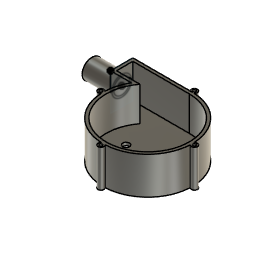
Bottom v3 (Autodesk Fusion 360 design; units mm, degrees)
Autodesk Fusion 360 part; units mm, degrees
sketch "Skizze1" plane through (0, 0, 0) normal (0, 0, 1) x (1, 0, 0)
  circle A0 centre (0, 0) radius 30
  circle A1 centre (0, 0) radius 3
  line L0 (0, 0) -> (14.5, 0)
  circle A2 centre (14.5, 0) radius 2.25
  line L1 (0, 0) -> (-14.5, 0)
  circle A3 centre (-14.5, 0) radius 2.25
  circle A4 centre (-31.5, 0) radius 1
  circle A5 centre (-31.5, 0) radius 2
  circle A6 centre (31.5, 0) radius 1
  circle A7 centre (31.5, 0) radius 2
  circle A8 centre (0, -31.5) radius 1
  circle A9 centre (0, -31.5) radius 2
  circle A10 centre (0, 31.5) radius 1
  circle A11 centre (0, 31.5) radius 2
  line L2 (0, 30) -> (-40, 30)
  line L3 (-40, 30) -> (-40, 15)
  line L4 (-40, 15) -> (0, 15)
  line L5 (0, 15) -> (0, 30)
  line L6 (-40, 30) -> (-40, 28)
  line L7 (-40, 28) -> (0, 28)
  circle A12 centre (0, 0) radius 28
  line L8 (-40, 15) -> (-40, 17)
  line L9 (-40, 17) -> (0, 17)
  line L10 (-38, 28) -> (-38, 17)
  dimension "d1" = 60
  dimension "d2" = 6
  dimension "d3" = 14.5
  dimension "d4" = 4.5
  dimension "d5" = 14.5
  dimension "d6" = 4.5
  dimension "d7" = 2
  dimension "d8" = 4
  dimension "d9" = 2
  dimension "d10" = 4
  dimension "d11" = 2
  dimension "d12" = 4
  dimension "d13" = 2
  dimension "d14" = 4
  dimension "d15" = 40
  dimension "d16" = 15
  dimension "d17" = 2
  dimension "d20" = 56
  dimension "d23" = 2
  constraint coincident A0.centre A1.centre
  constraint concentric A0 A1
  constraint horizontal L0
  constraint coincident L0.end A2.centre
  constraint parallel L0 L1
  constraint coincident L1.end A3.centre
  constraint concentric A4 A5
  constraint concentric A6 A7
  constraint concentric A8 A9
  constraint concentric A10 A11
  constraint horizontal L2
  constraint vertical L3
  constraint horizontal L4
  constraint vertical L5
  constraint coincident A0 L2.start
  constraint perpendicular L2 L6
  constraint coincident L5 L7.end
  constraint perpendicular L5 L7
  constraint concentric A1 A12
  constraint perpendicular L4 L8
  constraint coincident L5 L9.end
  constraint perpendicular L5 L9
  constraint coincident L7 L10.start
  constraint coincident L9 L10.end
  constraint perpendicular L9 L10
  measures "d1" diameter of A0
  measures "d2" diameter of A1
  measures "d3" distance of A0.centre L0.end
  measures "d4" diameter of A2
  measures "d5" distance of A0.centre L1.end
  measures "d6" diameter of A3
  measures "d7" diameter of A4
  measures "d8" diameter of A5
  measures "d9" diameter of A6
  measures "d10" diameter of A7
  measures "d11" diameter of A8
  measures "d12" diameter of A9
  measures "d13" diameter of A10
  measures "d14" diameter of A11
  measures "d15" distance of L2.start L2.end
  measures "d16" distance of L2.start L4.end
  measures "d17" distance of L2.end L6.end
  measures "d20" diameter of A12
  measures "d23" distance of L3.end L8.end
extrude "Extrusion1" add sketch "Skizze1" along normal blind 2 contours A0 A7 | A0 A5 A7 A9 A11 L4 L5 A12 | A0 A11 L5 | A0 A9 | A0 A11 L5 | A0 A11 L5 L7 | L4 L5 A12 | A0 L7 A12 L9 | L5 A12 L9 | A0 A5 | A0 L7 L9 L10 | L4 L5 A12 L9 | A0 L4 A12 L9 | L3 L7 L9 L10 picked at (29.8389, -0.2367) picked at (0, -29.8313) picked at (-29.8313, 0) makes body 1
extrude "Extrusion2" add sketch "Skizze1" along normal blind 25 contours A0 A7 | A0 A7 | A0 A5 A7 A9 A11 L4 L5 A12 | A0 A11 L5 | A0 A11 L2 | A0 A9 | A0 A9 | A0 A11 L5 | A0 A11 L5 L7 | A0 A5 | A0 A5 | A0 L4 A12 L9 picked at (-0.5627, 30.1897) bodies 1
extrude "Extrusion3" add sketch "Skizze1" along normal blind 25 contours A0 A11 L2 L3 L6 L7 | A0 L3 L4 L8 L9 | L3 L7 L9 L10 bodies 1
sketch "Skizze2" plane through (-40, 0, 0) normal (-1, 0, 0) x (0, -1, 0)
  line L0 (-30, 0) -> (-15, 0)
  line L1 (-15, 0) -> (-15, 25)
  line L2 (-15, 25) -> (-30, 25)
  line L3 (-30, 25) -> (-30, 0)
  line L4 (-15, 25) -> (-15, 12.5)
  line L5 (-15, 12.5) -> (-22.5, 12.5)
  circle A0 centre (-22.5, 12.5) radius 5.375
  circle A1 centre (-22.5, 12.5) radius 6.625
  dimension "d26" = 7.5
  dimension "d27" = 10.75
  dimension "d28" = 13.25
  constraint coincident L1.end L2.start
  constraint midpoint L1 L4.end
  constraint perpendicular L3 L5
  constraint coincident L5.end A0.centre
  constraint concentric A0 A1
  measures "d26" distance of L4.end L5.end
  measures "d27" diameter of A0
  measures "d28" diameter of A1
extrude "Extrusion4" cut sketch "Skizze2" against normal blind 2 contours A0 bodies 1
extrude "Extrusion5" add sketch "Skizze2" along normal blind 20 separate body contours A1 makes body 2
